Autodesk Inventor part; units mm, degrees
(part 2 of 2)
extrude "擠出6" add sketch "草圖2" along normal blind 3 contours A0 L70 A102 A101 A100 A496 A99 A98 A97 A96 A95 A94 L8 A93 A92 A91 A90 A89 A495 A88 A87 A86 A85 A84 A83 L7 A82 A81 A80 A79 A78 A494 A77 A76 A75 A74 A73 A72 L6 A71 A70 A69 A68 A67 A493 A66 A65 A64 A63 A62 A61 L5 A60 A59 A58 A57 A56 A506 A55 A54 A53 A52 A51 A50 L4 A49 A48 A47 A46 A45 A505 A44 A43 A42 A41 A40 A39 L3 A38 A37 A36 A35 A34 A504 A33 A32 A31 A30 A29 A28 L2 A27 A26 A25 A24 | A0 L70 A24 A23 A503 A22 A21 A20 A19 A18 A17 L1 A16 A15 A14 A13 A12 A502 A11 A10 A9 A8 A7 A6 L0 A5 A4 A3 A2 A1 A501 A155 A154 A153 A152 A151 A150 L13 A149 A148 A147 A146 A145 A500 A144 A143 A142 A141 A140 A139 L12 A138 A137 A136 A135 A134 A499 A133 A132 A131 A130 A129 A128 L11 A127 A126 A125 A124 A123 A498 A122 A121 A120 A119 A118 A117 L10 A116 A115 A114 A113 A112 A497 A111 A110 A109 A108 A107 A106 L9 A105 A104 A103 A102
extrude "擠出7" add sketch "草圖2" along normal blind 3 separate body contours A401 A402 A403 A404 A405 A406 A407 A408 A531 A409 A410 A411 A412 A413 A414 A415 A416 A417 A418 A419 A420 A530 A421 A422 A423 A424 A425 A426 A427 A428 A429 A430 A431 A432 A529 A433 A434 A435 A436 A437 A438 A439 A440 A441 A442 A443 A444 A528 A445 A446 A447 A448 A449 A450 A451 A452 A453 A454 A455 A456 A527 A457 A458 A459 A460 A461 A462 A463 A464 A465 A466 A467 A468 A526 A469 A470 A471 A472 A473 A474 A475 A476 A477 A478 A479 A480 A525 A481 A482 A483 A484 A485 A486 A487 A488 A489 A490 A491 A492 A524 A157 A158 A159 A160 A161 A162 A163 A164 A165 A166 A167 A168 A523 A169 A170 A171 A172 A173 A174 A175 A176 A177 A178 A179 A180 A522 A181 A182 A183 A184 A185 A186 A187 A188 A189 A190 A191 A192 A521 A193 A194 A195 A196 A197 A198 A199 A200 A201 A202 A203 A204 A520 A205 A206 A207 A208 A209 A210 A211 A212 A213 A214 A215 A216 A519 A217 A218 A219 A220 A221 A222 A223 A224 A225 A226 A227 A228 A518 A229 A230 A231 A232 A233 A234 A235 A236 A237 A238 A239 A240 A517 A241 A242 A243 A244 A245 A246 A247 A248 A249 A250 A251 A252 A516 A253 A254 A255 A256 A257 A258 A259 A260 A261 A262 A263 A264 A515 A265 A266 A267 A268 A269 A270 A271 A272 A273 A274 A275 A276 A514 A277 A278 A279 A280 A281 A282 A283 A284 A285 A286 A287 A288 A513 A289 A290 A291 A292 A293 A294 A295 A296 A297 A298 A299 A300 A512 A301 A302 A303 A304 A305 A306 A307 A308 A309 A310 A311 A312 A511 A313 A314 A315 A316 A317 A318 A319 A320 A321 A322 A323 A324 A510 A325 A326 A327 A328 A329 A330 A331 A332 A333 A334 A335 A336 A509 A337 A338 A339 A340 A341 A342 A343 A344 A345 A346 A347 A348 A508 A349 A350 A351 A352 A353 A354 A355 A356 A357 A358 A359 A360 A507 A361 A362 A363 A364 A365 A366 A367 A368 A369 A370 A371 A372 A534 A373 A374 A375 A376 A377 A378 A379 A380 A381 A382 A383 A384 A533 A385 A386 A387 A388 A389 A390 A391 A392 A393 A394 A395 A396 A532 A397 A398 A399 A400
